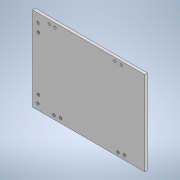
# Autodesk Inventor part: rightside new
Saved by Autodesk Inventor 2021.3 (Build 253353000, 353)
## iProperties
Created: 2021-07-01
Part Number: rightside new
Material: Generic
Document SubType Name: Modeling
Designer: Vijay
Density: 1 g/cm^3
Appearance: Default
Author: Vijay
Autodesk Inventor part; units mm, degrees
ref_plane "YZ Plane" through (0, 0, 0) normal (1, 0, 0) x (0, 1, 0)
ref_plane "XZ Plane" through (0, 0, 0) normal (0, 1, 0) x (-1, 0, 0)
ref_plane "XY Plane" through (0, 0, 0) normal (0, 0, 1) x (1, 0, 0)
sketch "Sketch1" plane through (0, 0, 0) normal (0, 0, 1) x (1, 0, 0)
  line L0 (-200, 150) -> (200, 150)
  line L1 (200, 150) -> (200, -150)
  line L2 (200, -150) -> (-200, -150)
  line L3 (-200, -150) -> (-200, 150)
  line L4 (-200, 150) -> (200, -150) construction
  line L5 (200, 150) -> (-200, -150) construction
  point P0 (0, 0)
  dimension "d0" = 400
  dimension "d1" = 300
  constraints: 12 end point, 2 midpoint, 2 parallel, 1 horizontal, 1 perpendicular
  measures "d0" distance of L1.end L2.end
  measures "d1" distance of L0.end L1.end
extrude "Extrusion1" add sketch "Sketch1" along normal blind 10
sketch "Sketch2" plane through (0, 0, 10) normal (0, 0, 1) x (1, 0, 0)
  point P0 (0, 0)
  point P1 (-179.2453, 119.35)
  point P2 (-178.3645, 91.164)
  point P3 (-178.3645, -100.853)
  point P4 (-180.1261, -129.039)
  point P5 (-138.7279, 136.0855)
  point P6 (-119.35, 135.2046)
  point P7 (93.8065, 137.8471)
  point P8 (116.7076, 137.8471)
  point P9 (-122.8733, -136.0855)
  point P10 (-99.0914, -133.443)
  point P11 (105.257, -136.9663)
  point P12 (128.1582, -134.3238)
hole "Hole1" at (-179.2453, 119.35, 10) at (-178.3645, 91.164, 10) at (-178.3645, -100.853, 10) at (-180.1261, -129.039, 10) at (-138.7279, 136.0855, 10) at (-119.35, 135.2046, 10) at (93.8065, 137.8471, 10) at (116.7076, 137.8471, 10) at (-122.8733, -136.0855, 10) at (-99.0914, -133.443, 10) at (105.257, -136.9663, 10) at (128.1582, -134.3238, 10) direction (0, 0, -1) diameter 9 end through all
body "Solid1"
